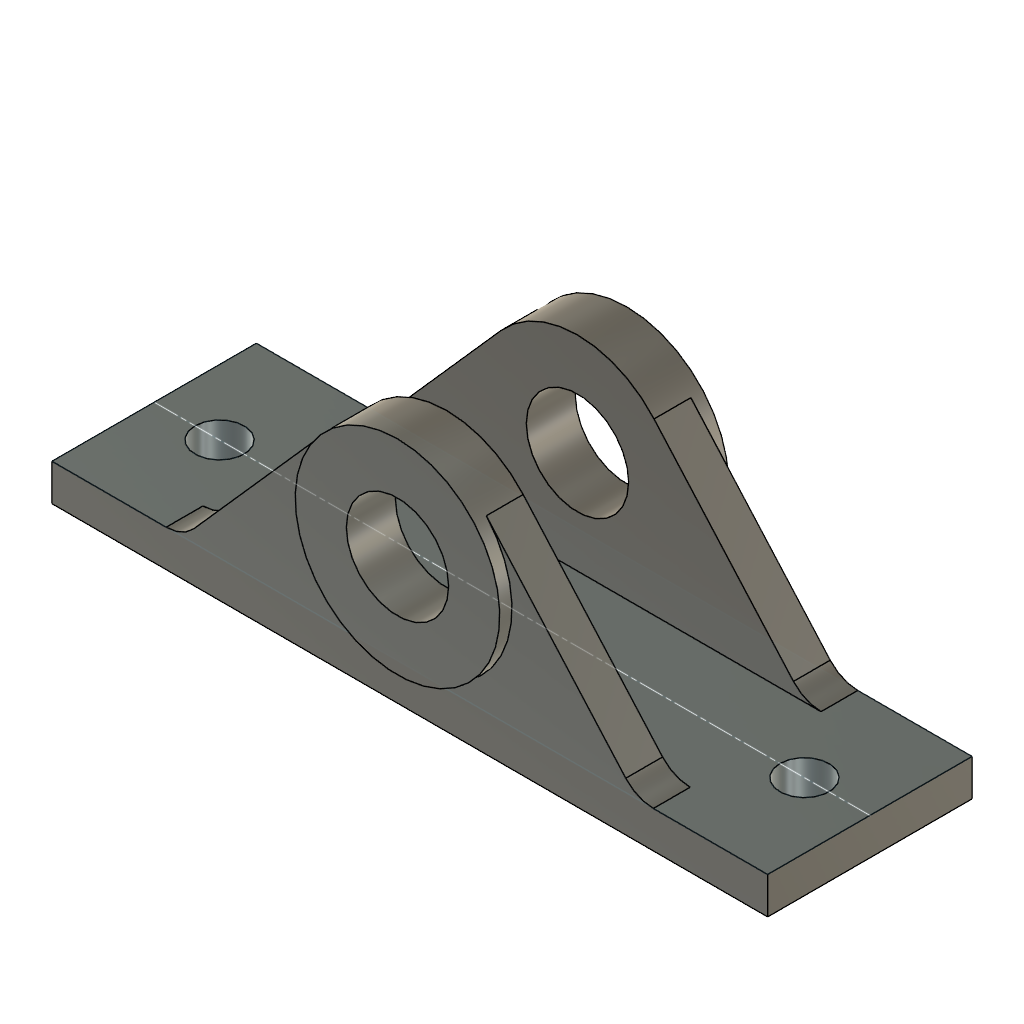
fusion exercise 2 (Autodesk Fusion 360 design; units mm, degrees)
part number: 2026-09-22-16-21-58-421
Autodesk Fusion 360 part; units mm, degrees
note: some values were not read from the file. Set by a fixed rule: which sketch regions a step uses.
sketch "Sketch1" plane through (0, 0, 0) normal (0, 0, 1) x (1, 0, 0)
  line L0 (87.5, 25) -> (-87.5, 25)
  line L1 (-87.5, 25) -> (-87.5, -25)
  line L2 (-87.5, -25) -> (87.5, -25)
  line L3 (87.5, -25) -> (87.5, 25)
  line L4 (87.5, 25) -> (-87.5, -25) construction
  line L5 (-87.5, 25) -> (87.5, -25) construction
  circle A0 centre (-71.5, 0) radius 6
  line L6 (0, 25) -> (0, -25) construction
  circle A1 centre (71.5, 0) radius 6
  dimension "d1" = 175
  dimension "d2" = 50
  dimension "d3" = 12
  dimension "d4" = 16
  dimension "d5" = 25
  constraint horizontal L0
  constraint perpendicular L0 L1
  constraint parallel L0 L2
  constraint parallel L1 L3
  constraint coincident L4 origin
  constraint coincident L5 origin
  constraint midpoint L0 L6.start
  constraint midpoint L2 L6.end
  constraint symmetric A0 L6 A1
  measures "d1" distance of L1.end L2.end
  measures "d2" distance of L0.end L1.end
  measures "d3" diameter of A0
  measures "d4" distance of L1 A0.centre
  measures "d5" distance of L2 A0.centre
extrude "Extrude1" add sketch "Sketch1" along normal blind 9 makes body 1
sketch "Sketch2" plane through (0, -25, 0) normal (0, -1, 0) x (1, 0, 0)
  line L0 (-87.5, 0) -> (87.5, 0)
  line L1 (87.5, 0) -> (87.5, 9)
  line L2 (87.5, 9) -> (-87.5, 9)
  line L3 (-87.5, 9) -> (-87.5, 0)
  line L4 (0, 9) -> (0, 34) construction
  circle A0 centre (0, 34) radius 25
  line L5 (-87.5, 9) -> (-55.5, 9) construction
  line L6 (87.5, 9) -> (55.5, 9) construction
  line L7 (-55.5, 9) -> (-18.7234, 50.566)
  line L8 (55.5, 9) -> (18.7234, 50.566)
  circle A1 centre (0, 34) radius 12.5
  dimension "d8" = 25
  dimension "d9" = 32
  dimension "d10" = 25
  constraint midpoint L2 L4.start
  constraint perpendicular L2 L4
  constraint coincident L4.end A0.centre
  constraint coincident L4.start A0
  constraint coincident L2.end L3.start
  constraint perpendicular L3 L5
  constraint symmetric L4 L2.end L1.end
  constraint symmetric L4 L5.end L6.end
  constraint coincident A0 L7.end
  constraint tangent A0 L7
  constraint symmetric L4 L7.end L8.end
  measures "d8" distance of L4.start L4.end
  measures "d9" distance of L2.end L5.end
  measures "d10" diameter of A1
sketch "Sketch3" plane through (0, 0, 9) normal (0, 0, 1) x (-1, 0, 0)
  circle A0 centre (71.5, 0) radius 6
  circle A1 centre (-71.5, 0) radius 6
  line L0 (-87.5, 25) -> (-87.5, -25)
  line L1 (-87.5, -25) -> (87.5, -25)
  line L2 (87.5, -25) -> (87.5, 25)
  line L3 (87.5, 25) -> (-87.5, 25)
  line L4 (-87.5, 0) -> (87.5, 0)
  constraint midpoint L0 L4.start
  constraint midpoint L2 L4.end
extrude "Extrude2" add sketch "Sketch2" against normal blind 9 separate body contours L2 A0 L7 | L2 A0 L8 | A0 makes body 2
sketch "Sketch4" plane through (0, -25, 0) normal (0, -1, 0) x (1, 0, 0)
  circle A0 centre (0, 34) radius 12.5
  line L0 (-55.5, 9) -> (55.5, 9)
  line L1 (55.5, 9) -> (18.7234, 50.566)
  arc A1 (18.7234, 50.566) -> (-18.7234, 50.566) centre (0, 34) ccw
  line L2 (-18.7234, 50.566) -> (-55.5, 9)
  circle A2 centre (0, 34) radius 25
  dimension "d13" = 50
  constraint concentric A0 A2
  measures "d13" diameter of A2
extrude "Extrude3" add sketch "Sketch4" along normal blind 3 contours A1 A2 bodies 1 2
sketch "Sketch5" plane through (0, 25, 0) normal (0, 1, 0) x (-1, 0, 0)
  line L0 (-87.5, 0) -> (87.5, 0)
  line L1 (87.5, 0) -> (87.5, 9)
  line L2 (87.5, 9) -> (-87.5, 9)
  line L3 (-87.5, 9) -> (-87.5, 0)
  circle A0 centre (0, 34) radius 12.5
  line L4 (-55.5, 9) -> (-18.7234, 50.566)
  line L5 (55.5, 9) -> (18.7234, 50.566)
  arc A1 (18.7234, 50.566) -> (-18.7234, 50.566) centre (0, 34) ccw
  line L6 (55.5, 9) -> (18.7234, 50.566)
  line L7 (87.5, 9) -> (55.5, 9)
  line L8 (87.5, 0) -> (87.5, 9)
  line L9 (87.5, 0) -> (-87.5, 0)
  line L10 (-87.5, 0) -> (-87.5, 9)
  line L11 (-55.5, 9) -> (-87.5, 9)
  line L12 (-55.5, 9) -> (-18.7234, 50.566)
  circle A2 centre (0, 34) radius 12.5
  arc A3 (18.7234, 50.566) -> (-18.7234, 50.566) centre (0, 34) ccw
  line L13 (87.5, 9) -> (55.5, 9)
  line L14 (87.5, 0) -> (87.5, 9)
  line L15 (87.5, 0) -> (-87.5, 0)
  line L16 (-87.5, 0) -> (-87.5, 9)
  line L17 (-55.5, 9) -> (-87.5, 9)
extrude "Extrude4" add sketch "Sketch5" against normal blind 9 contours L2 L4 L5 A1 L6 L12 A3 bodies 1
sketch "Sketch6" plane through (0, 25, 0) normal (0, 1, 0) x (-1, 0, 0)
  circle A0 centre (0, 34) radius 12.5
  line L0 (-87.5, 0) -> (87.5, 0)
  line L1 (87.5, 0) -> (87.5, 9)
  line L2 (87.5, 9) -> (55.5, 9)
  line L3 (55.5, 9) -> (18.7234, 50.566)
  arc A1 (18.7234, 50.566) -> (-18.7234, 50.566) centre (0, 34) ccw
  line L4 (-18.7234, 50.566) -> (-55.5, 9)
  line L5 (-55.5, 9) -> (-87.5, 9)
  line L6 (-87.5, 9) -> (-87.5, 0)
  circle A2 centre (0, 34) radius 25
  dimension "d18" = 50
  constraint concentric A0 A2
  measures "d18" diameter of A2
extrude "Extrude5" add sketch "Sketch6" along normal blind 3 contours A1 A2 bodies 1
fillet "Fillet1" radius 9 4 edges at (-55.5, -20.5, 9) (-55.5, 20.5, 9) (55.5, -20.5, 9) (55.5, 20.5, 9) on bodies 1
